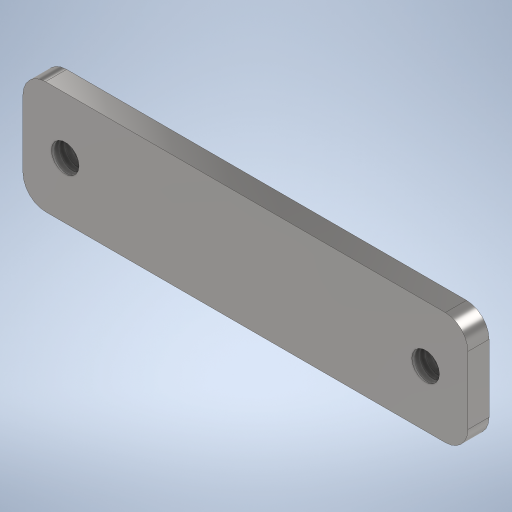
# Autodesk Inventor part: Cowling Magnetic Catch
Saved by Autodesk Inventor 2024 (Build 280153000, 153)
## iProperties
Created: 2023-06-20
Part Number: Cowling Magnetic Catch
Material: Steel, Carbon
Document SubType Name: Modeling
Designer: Ishaan
Density: 7.85 g/cm^3
Appearance: Semi-Polished
Author: Ishaan
Autodesk Inventor part; units mm, degrees
ref_plane "YZ Plane" through (0, 0, 0) normal (1, 0, 0) x (0, 1, 0)
ref_plane "XZ Plane" through (0, 0, 0) normal (0, 1, 0) x (-1, 0, 0)
ref_plane "XY Plane" through (0, 0, 0) normal (0, 0, 1) x (1, 0, 0)
sketch "Sketch1" plane through (0, 0, 0) normal (0, 0, 1) x (1, 0, 0)
  line L0 (19.75, -5) -> (-19.75, -5)
  line L1 (-19.75, -5) -> (-19.75, 5)
  line L2 (-19.75, 5) -> (19.75, 5)
  line L3 (19.75, 5) -> (19.75, -5)
  line L4 (19.75, -5) -> (-19.75, 5) construction
  line L5 (-19.75, -5) -> (19.75, 5) construction
  line L6 (16, 0) -> (-16, 0) construction
  point P0 (0, 0)
  point P1 (0, 5)
  point P2 (0, 0)
  dimension "d0" = 39.5
  dimension "d1" = 10
  dimension "d6" = 32
  constraints: 14 end point, 4 coincident, 4 midpoint, 2 horizontal, 2 parallel, 1 perpendicular, 1 vertical alignment
  measures "d0" distance of L1.end L2.end
  measures "d1" distance of L2.end L0.start
  measures "d6" distance of L6.start L6.end
extrude "Extrusion1" add sketch "Sketch1" along normal blind 1.8796
fillet "Fillet1" radius 2 4 edges at (-19.75, 5, 0.9398) (-19.75, -5, 0.9398) (19.75, -5, 0.9398) (19.75, 5, 0.9398)
hole "Hole1" at (16, 0, 0) at (-16, 0, 0) direction (0, 0, 1) diameter 2.459 end through all thread size "M3x0.5" class "6H" standard "ANSI Metric M Profile"
body "Solid1"
